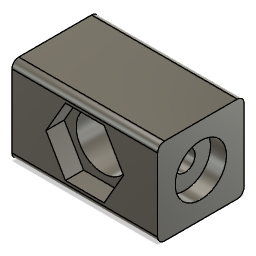
Hose Nozzle Holder v7 (Autodesk Fusion 360 design; units mm, degrees)
Autodesk Fusion 360 part; units mm, degrees
sketch "Sketch1" plane through (0, 0, 0) normal (0, 0, 1) x (1, 0, 0)
  line L0 (0, 25) -> (64, 25)
  line L1 (64, 25) -> (64, -13)
  line L2 (64, -13) -> (0, -13)
  line L3 (0, -13) -> (0, 25)
  dimension "d1" = 64
  dimension "d2" = 38
  constraint horizontal L0
  constraint vertical L1
  constraint horizontal L2
  constraint vertical L3
  measures "d1" distance of L0.start L0.end
  measures "d2" distance of L0.start L2.end
extrude "Extrude1" add sketch "Sketch1" along normal blind 38
sketch "Sketch2" plane through (0, 0, 38) normal (0, 0, 1) x (1, 0, 0)
  line L0 (0, -13) -> (64, -13)
  line L1 (64, -13) -> (64, 25)
  line L2 (64, 25) -> (0, 25)
  line L3 (0, 25) -> (0, -13)
  line L4 (0, 25) -> (64, -13) construction
  line L5 (40.5159, 20.75) -> (23.4841, 20.75)
  line L6 (23.4841, 20.75) -> (14.9682, 6)
  line L7 (14.9682, 6) -> (23.4841, -8.75)
  line L8 (23.4841, -8.75) -> (40.5159, -8.75)
  line L9 (40.5159, -8.75) -> (49.0318, 6)
  line L10 (49.0318, 6) -> (40.5159, 20.75)
  circle A0 centre (32, 6) radius 11.75
  point P0 (32, 6)
  point P1 (32, 6)
  dimension "d5" = 14.75
  dimension "d8" = 23.5
  constraint coincident L2.end L3.start
  constraint coincident L0.end L1.start
  constraint midpoint L4 P1
  constraint coincident P1 P0
  constraint parallel L2 L5
  measures "d5" distance of P1 L10
  measures "d8" diameter of A0
extrude "Extrude2" cut sketch "Sketch2" against normal blind 8 contours L5 L6 L7 L8 L9 L10 | A0
extrude "Extrude3" cut sketch "Sketch2" against normal blind 52 contours A0
sketch "Sketch4" plane through (0, 0, 0) normal (-1, 0, 0) x (0, 0, 1)
  line L0 (0, 25) -> (0, -13)
  line L1 (0, -13) -> (38, -13)
  line L2 (38, -13) -> (38, 25)
  line L3 (38, 25) -> (0, 25)
  circle A0 centre (19, 6) radius 6.75 construction
  line L4 (2.0294, 22.9706) -> (35.9706, -10.9706) construction
  line L5 (19, 25) -> (19, -13) construction
  line L6 (2.0294, -10.9706) -> (35.9706, 22.9706) construction
  line L7 (2.0294, 22.9706) -> (11.3071, 6)
  line L8 (2.0294, 22.9706) -> (19, 13.6929)
  line L9 (35.9706, 22.9706) -> (19, 13.6929)
  line L10 (35.9706, 22.9706) -> (26.6929, 6)
  line L11 (35.9706, -10.9706) -> (26.6929, 6)
  line L12 (35.9706, -10.9706) -> (19, -1.6929)
  line L13 (2.0294, -10.9706) -> (19, -1.6929)
  line L14 (2.0294, -10.9706) -> (11.3071, 6)
  line L15 (19, 6) -> (2.0294, 22.9706) construction
  line L16 (8.5702, 16.4298) -> (10.5147, 18.3317) construction
  line L17 (9.5, 15.5) -> (11.6895, 17.6895) construction
  line L18 (11.3986, 13.6014) -> (14.1445, 16.3473) construction
  line L19 (12.8128, 12.1872) -> (15.9732, 15.3476) construction
  line L20 (9.5, 15.5) -> (28.5, 15.5) construction
  line L21 (28.5, 15.5) -> (28.5, -3.5) construction
  line L22 (28.5, -3.5) -> (9.5, -3.5) construction
  line L23 (9.5, -3.5) -> (9.5, 15.5) construction
  line L24 (28.5, 15.5) -> (9.5, -3.5) construction
  circle A1 centre (9.5, 15.5) radius 1
  circle A2 centre (28.5, 15.5) radius 1
  circle A3 centre (28.5, -3.5) radius 1
  circle A4 centre (9.5, -3.5) radius 1
  point P0 (19, 6)
  point P1 (12.8128, 12.1872)
  point P2 (11.3986, 13.6014)
  point P3 (9.5, 15.5)
  point P4 (8.5702, 16.4298)
  point P5 (14.227, 10.773)
  point P6 (28.5, 15.5)
  point P7 (9.5, -3.5)
  point P8 (28.5, -3.5)
  dimension "d11" = 13.5
  dimension "d12" = 48
  dimension "d13" = 48
  dimension "d33" = 19
  dimension "d34" = -19
  dimension "d35" = 2
  dimension "d36" = 2
  dimension "d37" = 2
  dimension "d38" = 2
  constraint coincident P0 A0.centre
  constraint midpoint L3 L5.start
  constraint midpoint L1 L5.end
  constraint midpoint P0 L5
  constraint midpoint P0 L4
  constraint perpendicular L4 L6
  constraint midpoint P0 L6
  constraint tangent A0 L7
  constraint tangent A0 L8
  constraint tangent A0 L9
  constraint tangent A0 L10
  constraint tangent A0 L11
  constraint tangent A0 L12
  constraint tangent A0 L13
  constraint tangent A0 L14
  constraint coincident L5 L8.end
  constraint coincident L5 L12.end
  constraint coincident L4 P1
  constraint coincident L15 P2
  constraint coincident L15 P3
  constraint coincident L15 P4
  constraint coincident A0 P5
  constraint coincident L4 P5
  constraint coincident P4 L16.start
  constraint midpoint L8 L16.end
  constraint coincident P3 L17.start
  constraint coincident L8 L17.end
  constraint perpendicular L4 L17
  constraint coincident P2 L18.start
  constraint coincident L8 L18.end
  constraint perpendicular L15 L18
  constraint coincident P1 L19.start
  constraint coincident L8 L19.end
  constraint perpendicular L15 L19
  constraint horizontal L20
  constraint vertical L21
  constraint horizontal L22
  constraint vertical L23
  constraint coincident P8 L21.end
  constraint coincident P6 L20.end
  constraint coincident P7 L22.end
  constraint midpoint P0 L24
  measures "d11" diameter of A0
  measures "d12" distance of L4.start L4.end
  measures "d13" distance of L6.start L6.end
  measures "d35" diameter of A1
  measures "d36" diameter of A4
  measures "d37" diameter of A3
  measures "d38" diameter of A2
extrude "Extrude4" cut sketch "Sketch4" against normal blind 3 contours L7 L8 L9 L10 L11 L12 L13 L14 | A1 | A2 | A3 | A4
fillet "Fillet1" radius 3 2 edges at (32, 25, 0) (32, -13, 0)
fillet "Fillet2" radius 3 2 edges at (32, 25, 38) (32, -13, 38)
sketch "Sketch5" plane through (64, 0, 0) normal (1, 0, 0) x (0, 0, -1)
  arc A0 (-38, -10) -> (-35, -13) centre (-35, -10) ccw
  line L0 (-35, -13) -> (-3, -13)
  arc A1 (-3, -13) -> (0, -10) centre (-3, -10) ccw
  line L1 (0, -10) -> (0, 22)
  arc A2 (0, 22) -> (-3, 25) centre (-3, 22) ccw
  line L2 (-3, 25) -> (-35, 25)
  arc A3 (-35, 25) -> (-38, 22) centre (-35, 22) ccw
  line L3 (-38, 22) -> (-38, -10)
  circle A4 centre (-19, 6) radius 11.25
  circle A5 centre (-19, 6) radius 4.5
  point P0 (-19, 25)
  point P1 (-19, -13)
  point P2 (-38, 6)
  point P3 (0, 6)
  point P4 (-19, 6)
  dimension "d20" = 22.5
  dimension "d21" = 9
  constraint midpoint L2 P0
  constraint midpoint L0 P1
  constraint midpoint L3 P2
  constraint midpoint L1 P3
  constraint coincident P4 A4.centre
  measures "d20" diameter of A4
  measures "d21" diameter of A5
extrude "Extrude5" cut sketch "Sketch5" against normal blind 18 contours A5
extrude "Extrude6" cut sketch "Sketch5" against normal blind 7 contours A4
extrude "Extrude7" cut sketch "Sketch4" against normal blind 4 contours L7 L8 L9 L10 L11 L12 L13 L14 | A1 | A2 | A3 | A4
extrude "Extrude8" cut sketch "Sketch4" against normal blind 7 contours A1 | A2 | A3 | A4
